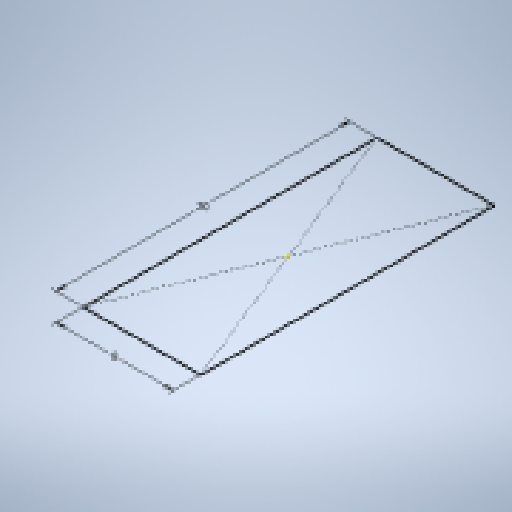
# Autodesk Inventor part: Base
Saved by Autodesk Inventor 2024 (Build 280153000, 153)
## iProperties
Created: 2023-08-25
Part Number: Base
Material: Genérico
Document SubType Name: Modeling
Designer: sergi
Density: 1 g/cm^3
Appearance: Valor por defecto
Author: sergi
Autodesk Inventor part; units mm, degrees
ref_plane "YZ Plane" through (0, 0, 0) normal (1, 0, 0) x (0, 1, 0)
ref_plane "XZ Plane" through (0, 0, 0) normal (0, 1, 0) x (-1, 0, 0)
ref_plane "XY Plane" through (0, 0, 0) normal (0, 0, 1) x (1, 0, 0)
sketch "Boceto1" plane through (0, 0, 0) normal (0, 1, 0) x (-1, 0, 0)
  line L0 (-6, -10) -> (6, -10)
  line L1 (6, -10) -> (6, 10)
  line L2 (6, 10) -> (-6, 10)
  line L3 (-6, 10) -> (-6, -10)
  line L4 (-6, -10) -> (6, 10) construction
  line L5 (6, -10) -> (-6, 10) construction
  point P0 (0, 0)
  dimension "d0" = 12
  dimension "d1" = 20
  constraints: 12 end point, 2 midpoint, 2 parallel, 1 horizontal, 1 perpendicular
  measures "d0" distance of L2.end L1.end
  measures "d1" distance of L1.end L0.end
extrude "Extrusión1" add sketch "Boceto1" along normal blind 12
fillet "Empalme1" radius 6 2 edges at (-6, 12, 0) (-6, 0, 0)
sketch "Boceto2" plane through (6, 0, -10) normal (0, 0, -1) x (-1, 0, 0)
  arc A0 (6, 0) -> (6, 12) centre (6, 6) ccw projected
  constraints: 1 coincident
hole "Agujero1" at (0, 6, -10) direction (0, 0, 1) diameter 4 depth 12 tip angle 118
sketch "Boceto3" plane through (6, 0, -10) normal (0, 0, -1) x (-1, 0, 0)
  circle A0 centre (6, 6) radius 2 projected
  line L0 (46.075, 3.0009) -> (6.1, 2.0013) projected
  arc A1 (46.075, 3.0009) -> (46.075, 8.9991) centre (46, 6) ccw projected
  line L1 (6.1, 9.9987) -> (46.075, 8.9991) projected
  arc A2 (6.1, 9.9987) -> (6.1, 2.0013) centre (6, 6) ccw projected
  circle A3 centre (6, 6) radius 2 projected
  arc A4 (6, 0) -> (6, 12) centre (6, 6) ccw projected
  line L2 (0, 12) -> (6, 12) projected
  line L3 (0, 0) -> (0, 12) projected
  line L4 (0, 0) -> (6, 0) projected
  line L5 (2, 6) -> (2, 13.7871)
  line L6 (1.5, 6) -> (1.5, 13.7871)
  line L7 (6.1125, 1.5014) -> (46.0875, 2.5011)
  arc A5 (46.0875, 2.5011) -> (46.0875, 9.4989) centre (46, 6) ccw
  line L8 (46.0875, 9.4989) -> (6.1125, 10.4986)
  arc A6 (6.1125, 10.4986) -> (6.1125, 1.5014) centre (6, 6) ccw
  point P0 (6, 0)
  point P1 (2, 12)
  point P2 (10.5707, 2.1131)
  point P3 (10.0799, 10.3994)
  point P4 (1.5, 12)
  dimension "d14" = 0.5
  dimension "d15" = 0.5
  constraints: 8 end point, 5 point on circle, 2 centre point, 1 parallel, 1 tangent, 1 vertical, 3 other
  measures "d14" distance between parallel lines of L5 L6
  measures "d15" radial gap between concentric circles of A2 A6
extrude "Extrusión2" cut sketch "Boceto3" against normal blind 7 contours A0 | A1 L1 A4 L8 A5 L7 L0 | L0 A4 L1 A1 | A4 L7 A6 L5 A2 L0 | L0 A2 L1 A4 | L1 A2 L5 A6 L8 A4 | L8 A6 L5 L2 A4 | A6 L6 L2 L5
mirror "Simetría1" about plane through (6, 0, -10) normal (0, 0, -1) remove original yes
